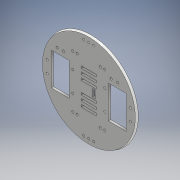
# Autodesk Inventor part: learnbotDown
Saved by Autodesk Inventor 2017 (Build 210142000, 142)
## iProperties
Part Number: learnbotDown
Material: Genérico
Document SubType Name: Modeling
Designer: rober
Density: 1 g/cm^3
Appearance: Valor por defecto
Author: rober
Autodesk Inventor part; units mm, degrees
ref_plane "YZ Plane" through (0, 0, 0) normal (1, 0, 0) x (0, 1, 0)
ref_plane "XZ Plane" through (0, 0, 0) normal (0, 1, 0) x (-1, 0, 0)
ref_plane "XY Plane" through (0, 0, 0) normal (0, 0, 1) x (1, 0, 0)
sketch "Boceto1" plane through (0, 0, 0) normal (0, 0, 1) x (1, 0, 0)
  arc A0 (-6.3439, 0.3) -> (-6.25, 0) centre (18.1956, 7.818) ccw
  line L0 (-6.25, 0) -> (0, 0)
  line L1 (0, 0) -> (0, 0.3)
  line L2 (0, 0.3) -> (-6.3439, 0.3)
  constraints: 6 end point, 2 point on circle, 1 centre point
revolve "Revolución1" add sketch "Boceto1" angle 360 about axis through (0, 0, 0) along (0, 1, 0)
sketch "Boceto2" plane through (0, 0.3, 0) normal (0, 1, 0) x (1, 0, 0)
  circle A0 centre (-0.0005, 5.6024) radius 0.15
  circle A1 centre (-5.6181, 0.8021) radius 0.15
  circle A2 centre (5.6033, 0.7979) radius 0.15
  circle A3 centre (0, 0) radius 6.25 projected
  circle A4 centre (-0.0005, -5.6024) radius 0.15
  circle A5 centre (-5.6181, -0.8021) radius 0.15
  circle A6 centre (5.6033, -0.7979) radius 0.15
  point P0 (-0.8, 0.7979)
  constraints: 6 centre point
extrude "Extrusión1" cut sketch "Boceto2" against normal blind 10 contours A0 | A1 | A2 | A4 | A5 | A6
sketch "Boceto5" plane through (0, 0.3, 0) normal (0, 1, 0) x (1, 0, 0)
  circle A0 centre (0, 0) radius 6.25
  line L0 (-5.05, 0) -> (-5.05, -2.2)
  line L1 (-5.05, -2.2) -> (-2.65, -2.2)
  line L2 (-2.65, -2.2) -> (-2.65, 2.2)
  line L3 (-2.65, 2.2) -> (-5.05, 2.2)
  line L4 (-5.05, 2.2) -> (-5.05, 0)
  line L5 (5.05, 0) -> (5.05, -2.2)
  line L6 (5.05, -2.2) -> (2.65, -2.2)
  line L7 (2.65, -2.2) -> (2.65, 2.2)
  line L8 (2.65, 2.2) -> (5.05, 2.2)
  line L9 (5.05, 2.2) -> (5.05, 0)
  circle A1 centre (-5.618, 0.796) radius 0.15
  circle A2 centre (-5.618, -0.796) radius 0.15
  circle A3 centre (5.618, 0.796) radius 0.15
  circle A4 centre (5.618, -0.796) radius 0.15
  circle A5 centre (-2.15, -1.394) radius 0.15
  circle A6 centre (-2.15, 1.394) radius 0.15
  circle A7 centre (2.15, -1.394) radius 0.15
  circle A8 centre (2.15, 1.394) radius 0.15
  circle A9 centre (0, -5.6) radius 0.15
  circle A10 centre (0, 5.6) radius 0.15
  line L10 (1, -0.7) -> (1, -1)
  line L11 (1, -1) -> (-1, -1)
  line L12 (-1, -1) -> (-1, -0.7)
  line L13 (-1, -0.7) -> (1, -0.7)
  line L14 (1, -1.4) -> (1, -1.7)
  line L15 (1, -1.7) -> (-1, -1.7)
  line L16 (-1, -1.7) -> (-1, -1.4)
  line L17 (-1, -1.4) -> (1, -1.4)
  line L18 (1, -2.1) -> (1, -2.4)
  line L19 (1, -2.4) -> (-1, -2.4)
  line L20 (-1, -2.4) -> (-1, -2.1)
  line L21 (-1, -2.1) -> (1, -2.1)
  line L22 (-1, 1) -> (-1, 0.7)
  line L23 (-1, 0.7) -> (1, 0.7)
  line L24 (1, 0.7) -> (1, 1)
  line L25 (1, 1) -> (-1, 1)
  line L26 (-1, 1.7) -> (-1, 1.4)
  line L27 (-1, 1.4) -> (1, 1.4)
  line L28 (1, 1.4) -> (1, 1.7)
  line L29 (1, 1.7) -> (-1, 1.7)
  line L30 (-1, 2.4) -> (-1, 2.1)
  line L31 (-1, 2.1) -> (1, 2.1)
  line L32 (1, 2.1) -> (1, 2.4)
  line L33 (1, 2.4) -> (-1, 2.4)
  circle A11 centre (-2.15, 3.55) radius 0.15
  circle A12 centre (-1.55, 3.55) radius 0.15
  circle A13 centre (2.15, 3.55) radius 0.15
  circle A14 centre (1.55, 3.55) radius 0.15
  circle A15 centre (-2.15, -3.55) radius 0.15
  circle A16 centre (-1.55, -3.55) radius 0.15
  circle A17 centre (2.15, -3.55) radius 0.15
  circle A18 centre (1.55, -3.55) radius 0.15
  line L34 (0.6, 0.4) -> (0.6, -0.4)
  line L35 (0.6, -0.4) -> (0.7, -0.4)
  line L36 (0.7, -0.4) -> (0.8, -0.3)
  line L37 (0.8, -0.3) -> (0.8, 0.3)
  line L38 (0.8, 0.3) -> (0.7, 0.4)
  line L39 (0.7, 0.4) -> (0.6, 0.4)
  line L40 (0.5, 0) -> (0.5, -0.5)
  line L41 (0.5, -0.5) -> (0.9, -0.5)
  line L42 (0.9, -0.5) -> (0.9, 0.5)
  line L43 (0.9, 0.5) -> (0.5, 0.5)
  line L44 (0.5, 0.5) -> (0.5, 0)
  constraints: 90 end point, 19 centre point
extrude "Extrusión4" cut sketch "Boceto5" against normal blind 10 contours L4 L3 L2 L1 L0 | L5 L6 L7 L8 L9 | A5 | A6 | A7 | A8 | L10 L11 L12 L13 | L14 L15 L16 L17 | L18 L19 L20 L21 | L25 L24 L23 L22 | L29 L28 L27 L26 | L33 L32 L31 L30 | A11 | A12 | A13 | A14 | A15 | A16 | A17 | A18 | L39 L38 L37 L36 L35 L34 | L44 L43 L42 L41 L40
sketch "Boceto8" plane through (0, 0.3, 0) normal (0, 1, 0) x (1, 0, 0)
  circle A0 centre (0, 0) radius 6.25
  line L0 (-5.05, 0) -> (-5.05, -2.2)
  line L1 (-5.05, -2.2) -> (-2.65, -2.2)
  line L2 (-2.65, -2.2) -> (-2.65, 2.2)
  line L3 (-2.65, 2.2) -> (-5.05, 2.2)
  line L4 (-5.05, 2.2) -> (-5.05, 0)
  line L5 (5.05, 0) -> (5.05, -2.2)
  line L6 (5.05, -2.2) -> (2.65, -2.2)
  line L7 (2.65, -2.2) -> (2.65, 2.2)
  line L8 (2.65, 2.2) -> (5.05, 2.2)
  line L9 (5.05, 2.2) -> (5.05, 0)
  circle A1 centre (-5.618, 0.796) radius 0.15
  circle A2 centre (-5.618, -0.796) radius 0.15
  circle A3 centre (5.618, 0.796) radius 0.15
  circle A4 centre (5.618, -0.796) radius 0.15
  circle A5 centre (-2.15, -1.394) radius 0.15
  circle A6 centre (-2.15, 1.394) radius 0.15
  circle A7 centre (2.15, -1.394) radius 0.15
  circle A8 centre (2.15, 1.394) radius 0.15
  circle A9 centre (0, -5.6) radius 0.15
  circle A10 centre (0, 5.6) radius 0.15
  line L10 (1, -0.7) -> (1, -1)
  line L11 (1, -1) -> (-1, -1)
  line L12 (-1, -1) -> (-1, -0.7)
  line L13 (-1, -0.7) -> (1, -0.7)
  line L14 (1, -1.4) -> (1, -1.7)
  line L15 (1, -1.7) -> (-1, -1.7)
  line L16 (-1, -1.7) -> (-1, -1.4)
  line L17 (-1, -1.4) -> (1, -1.4)
  line L18 (1, -2.1) -> (1, -2.4)
  line L19 (1, -2.4) -> (-1, -2.4)
  line L20 (-1, -2.4) -> (-1, -2.1)
  line L21 (-1, -2.1) -> (1, -2.1)
  line L22 (-1, 1) -> (-1, 0.7)
  line L23 (-1, 0.7) -> (1, 0.7)
  line L24 (1, 0.7) -> (1, 1)
  line L25 (1, 1) -> (-1, 1)
  line L26 (-1, 1.7) -> (-1, 1.4)
  line L27 (-1, 1.4) -> (1, 1.4)
  line L28 (1, 1.4) -> (1, 1.7)
  line L29 (1, 1.7) -> (-1, 1.7)
  line L30 (-1, 2.4) -> (-1, 2.1)
  line L31 (-1, 2.1) -> (1, 2.1)
  line L32 (1, 2.1) -> (1, 2.4)
  line L33 (1, 2.4) -> (-1, 2.4)
  circle A11 centre (-2.15, 3.55) radius 0.15
  circle A12 centre (-1.55, 3.55) radius 0.15
  circle A13 centre (2.15, 3.55) radius 0.15
  circle A14 centre (1.55, 3.55) radius 0.15
  circle A15 centre (-2.15, -3.55) radius 0.15
  circle A16 centre (-1.55, -3.55) radius 0.15
  circle A17 centre (2.15, -3.55) radius 0.15
  circle A18 centre (1.55, -3.55) radius 0.15
  line L34 (0.6, 0.4) -> (0.6, -0.4)
  line L35 (0.6, -0.4) -> (0.7, -0.4)
  line L36 (0.7, -0.4) -> (0.8, -0.3)
  line L37 (0.8, -0.3) -> (0.8, 0.3)
  line L38 (0.8, 0.3) -> (0.7, 0.4)
  line L39 (0.7, 0.4) -> (0.6, 0.4)
  line L40 (0.5, 0) -> (0.5, -0.5)
  line L41 (0.5, -0.5) -> (0.9, -0.5)
  line L42 (0.9, -0.5) -> (0.9, 0.5)
  line L43 (0.9, 0.5) -> (0.5, 0.5)
  line L44 (0.5, 0.5) -> (0.5, 0)
  circle A19 centre (3, -2.8935) radius 0.15
  circle A20 centre (3.9, -2.8935) radius 0.15
  circle A21 centre (-3.4, -2.8935) radius 0.15
  circle A22 centre (-4.25, -2.8935) radius 0.15
  circle A23 centre (-0.675, -5.6) radius 0.15
  circle A24 centre (0.675, -5.6) radius 0.15
  circle A25 centre (-0.675, 5.6) radius 0.15
  circle A26 centre (0.675, 5.6) radius 0.15
  constraints: 90 end point, 27 centre point
extrude "Extrusión7" cut sketch "Boceto8" against normal blind 10 contours A19 | A20 | A21 | A22 | A23 | A24 | A25 | A26
